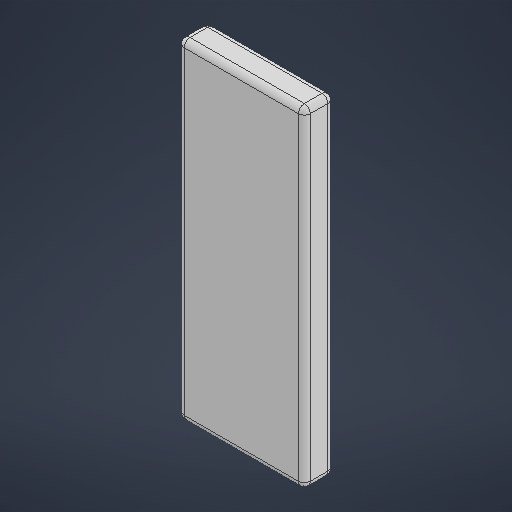
# Autodesk Inventor part: 上板电池
Saved by Autodesk Inventor 2025 (Build 290162000, 162)
## iProperties
Created: 2025-11-17
Part Number: 上板电池
Material: 常规
Document SubType Name: Modeling
Designer: XH
Density: 1 g/cm^3
Appearance: 默认
Author: XH
Autodesk Inventor part; units mm, degrees
ref_plane "YZ Plane" through (0, 0, 0) normal (1, 0, 0) x (0, 1, 0)
ref_plane "XZ Plane" through (0, 0, 0) normal (0, 1, 0) x (-1, 0, 0)
ref_plane "XY Plane" through (0, 0, 0) normal (0, 0, 1) x (1, 0, 0)
sketch "草图1" plane through (0, 0, 0) normal (0, 0, 1) x (1, 0, 0)
  line L0 (10.7, -28) -> (-10.7, -28)
  line L1 (-10.7, -28) -> (-10.7, 28)
  line L2 (-10.7, 28) -> (10.7, 28)
  line L3 (10.7, 28) -> (10.7, -28)
  line L4 (10.7, -28) -> (-10.7, 28) construction
  line L5 (-10.7, -28) -> (10.7, 28) construction
  point P0 (0, 0)
  dimension "d0" = 56
  dimension "d1" = 21.4
  constraints: 12 end point, 2 midpoint, 2 parallel, 1 horizontal, 1 perpendicular
  measures "d0" distance of L2.end L0.start
  measures "d1" distance of L1.end L2.end
extrude "拉伸1" add sketch "草图1" along normal blind 5
fillet "圆角1" radius 1 12 edges at (-10.7, 0, 5) (10.7, 0, 5) (0, 28, 5) (10.7, 28, 2.5) (0, 28, 0) (10.7, 0, 0) (-10.7, 0, 0) (-10.7, -28, 2.5) (10.7, -28, 2.5) (0, -28, 0) (0, -28, 5) (-10.7, 28, 2.5)
